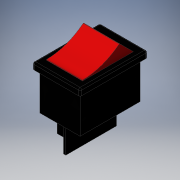
# Autodesk Inventor part: GRSV-4011-0137_RockerSwitch
Saved by Autodesk Inventor 2016 (Build 200138000, 138)
## iProperties
Created: 2016-09-24
Part Number: GRSV-4011-0137_RockerSwitch
Material: Generic
Document SubType Name: Modeling
Designer: jfixelle
Density: 1 g/cm^3
Appearance: Black
Author: jfixelle
Autodesk Inventor part; units mm, degrees
ref_plane "YZ Plane" through (0, 0, 0) normal (1, 0, 0) x (0, 1, 0)
ref_plane "XZ Plane" through (0, 0, 0) normal (0, 1, 0) x (-1, 0, 0)
ref_plane "XY Plane" through (0, 0, 0) normal (0, 0, 1) x (1, 0, 0)
sketch "Sketch1" plane through (0, 0, 0) normal (0, 1, 0) x (-1, 0, 0)
  line L0 (7.495, 10.605) -> (-7.495, 10.605)
  line L1 (-7.495, 10.605) -> (-7.495, -10.605)
  line L2 (-7.495, -10.605) -> (7.495, -10.605)
  line L3 (7.495, -10.605) -> (7.495, 10.605)
  point P0 (0, 0)
  dimension "d0" = 14.99
  dimension "d1" = 7.495
  dimension "d2" = 21.21
  dimension "d3" = 10.605
  constraints: 8 end point, 2 parallel, 1 horizontal, 1 perpendicular
  measures "d0" distance of L0.start L0.end
  measures "d1" distance from line of point (0, 0) L3
  measures "d2" distance of L2.end L0.start
  measures "d3" distance from line of point (0, 0) L2
extrude "Extrusion1" add sketch "Sketch1" against normal blind 2.03
sketch "Sketch2" plane through (0, -2.03, 0) normal (0, -1, 0) x (1, 0, 0)
  line L0 (-6.35, 9.46) -> (6.35, 9.46)
  line L1 (6.35, 9.46) -> (6.35, -9.46)
  line L2 (6.35, -9.46) -> (-6.35, -9.46)
  line L3 (-6.35, -9.46) -> (-6.35, 9.46)
  point P0 (0, 0)
  dimension "d6" = 12.7
  dimension "d7" = 6.35
  dimension "d8" = 18.92
  dimension "d9" = 9.46
  constraints: 8 end point, 2 parallel, 1 horizontal, 1 perpendicular
  measures "d6" distance of L0.start L0.end
  measures "d7" distance from line of point (0, 0) L1
  measures "d8" distance of L0.end L1.end
  measures "d9" distance from line of point (0, 0) L2
extrude "Extrusion2" add sketch "Sketch2" along normal blind 11.93
sketch "Sketch3" plane through (0, -13.96, 0) normal (0, -1, 0) x (1, 0, 0)
  line L0 (-0.38, -8) -> (0.38, -8)
  line L1 (0.38, -8) -> (0.38, 8)
  line L2 (0.38, 8) -> (-0.38, 8)
  line L3 (-0.38, 8) -> (-0.38, -8)
  point P0 (0, 0)
  dimension "d12" = 0.76
  dimension "d13" = 0.38
  dimension "d14" = 16
  dimension "d15" = 8
  constraints: 8 end point, 2 parallel, 1 horizontal, 1 perpendicular
  measures "d12" distance of L1.end L2.end
  measures "d13" distance from line of point (0, 0) L3
  measures "d14" distance of L0.end L1.end
  measures "d15" distance from line of point (0, 0) L2
extrude "Extrusion3" add sketch "Sketch3" along normal blind 8.89
fillet "Fillet1" radius 0.5 8 edges at (7.495, -1.015, -10.605) (7.495, 0, 0) (7.495, -1.015, 10.605) (0, 0, 10.605) (-7.495, -1.015, 10.605) (-7.495, 0, 0) (-7.495, -1.015, -10.605) (0, 0, -10.605)
sketch "Sketch4" plane through (0, -13.96, 0) normal (0, -1, 0) x (1, 0, 0)
  line L0 (-1.6, -6.675) -> (-6.35, -6.675)
  line L1 (-6.35, -6.675) -> (-6.35, -5.865)
  line L2 (-6.35, -5.865) -> (-1.6, -5.865)
  line L3 (-1.6, -5.865) -> (-1.6, -6.675)
  line L4 (-1.6, -0.405) -> (-6.35, -0.405)
  line L5 (-6.35, -0.405) -> (-6.35, 0.405)
  line L6 (-6.35, 0.405) -> (-1.6, 0.405)
  line L7 (-1.6, 0.405) -> (-1.6, -0.405)
  line L8 (-1.6, 3.145) -> (-6.35, 3.145)
  line L9 (-6.35, 3.145) -> (-6.35, 3.955)
  line L10 (-6.35, 3.955) -> (-1.6, 3.955)
  line L11 (-1.6, 3.955) -> (-1.6, 3.145)
  line L12 (-6.35, 9.46) -> (-6.35, -9.46) projected
  point P0 (0, 0)
  dimension "d19" = 0
  dimension "d20" = 4.75
  dimension "d21" = 4.75
  dimension "d22" = 0.81
  dimension "d23" = 0.81
  dimension "d24" = 0.81
  dimension "d25" = 5.46
  dimension "d26" = 2.74
  dimension "d28" = 0.405
  constraints: 24 end point, 6 parallel, 3 horizontal, 3 perpendicular, 3 point on line
  measures "d19" distance between parallel lines of L12 L1
  measures "d20" distance of L0.start L0.end
  measures "d21" distance of L9.end L10.end
  measures "d22" distance between parallel lines of L10 L8
  measures "d23" distance between parallel lines of L6 L4
  measures "d24" distance between parallel lines of L2 L0
  measures "d25" distance between parallel lines of L4 L2
  measures "d26" distance between parallel lines of L8 L6
  measures "d28" distance from line of point (0, 0) L4
extrude "Extrusion4" add sketch "Sketch4" along normal blind 8.38
sketch "Sketch5" plane through (0, 0, 0) normal (0, 1, 0) x (1, 0, 0)
  line L0 (5.65, 8) -> (-5.65, 8)
  line L1 (-5.65, 8) -> (-5.65, -8)
  line L2 (-5.65, -8) -> (5.65, -8)
  line L3 (5.65, -8) -> (5.65, 8)
  point P0 (0, 0)
  dimension "d31" = 16
  dimension "d32" = 8
  dimension "d33" = 11.3
  dimension "d34" = 5.65
  constraints: 8 end point, 2 parallel, 1 horizontal, 1 perpendicular
  measures "d31" distance of L2.end L0.start
  measures "d32" distance from line of point (0, 0) L2
  measures "d33" distance of L1.end L2.end
  measures "d34" distance from line of point (0, 0) L3
extrude "Extrusion5" add sketch "Sketch5" along normal blind 4.32
sketch "Sketch7" plane through (-5.65, 0, 8) normal (-1, 0, 0) x (0, 0, 1)
  circle A0 centre (0.1807, 19.0432) radius 18.7949
  point P0 (-8, 0)
  constraints: 1 centre point
extrude "Extrusion7" cut sketch "Sketch7" along normal through all both and the other way through all
chamfer "Chamfer1" distance 4.32 angle 45 1 edges at (0, 4.32, -8) measured on face at (1.8833, 2.88, -8)
body "Solid1"
